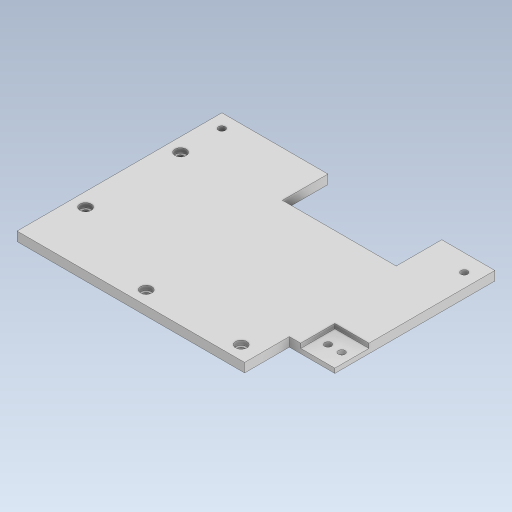
# Autodesk Inventor part: Casis Kanan Bawah
Saved by Autodesk Inventor 2023.5 (Build 275446000, 446)
## iProperties
Created: 2025-09-16
Part Number: Casis Kanan Bawah
Material: Generic
Document SubType Name: Modeling
Designer: Guntur
Density: 1 g/cm^3
Appearance: Default
Author: Guntur
Autodesk Inventor part; units mm, degrees
ref_plane "YZ Plane" through (0, 0, 0) normal (1, 0, 0) x (0, 1, 0)
ref_plane "XZ Plane" through (0, 0, 0) normal (0, 1, 0) x (-1, 0, 0)
ref_plane "XY Plane" through (0, 0, 0) normal (0, 0, 1) x (1, 0, 0)
sketch "Sketch1" plane through (0, 0, 0) normal (0, 1, 0) x (-1, 0, 0)
  circle A0 centre (-7.6905, 26.7159) radius 1.5
  circle A1 centre (-7.6905, 14.7159) radius 1.5
  line L0 (-0.1905, 5.7159) -> (-15.1905, 5.7159)
  line L1 (-15.1905, 35.7159) -> (-0.1905, 35.7159)
  line L2 (-15.1905, 5.7159) -> (-15.1905, 35.7159)
  circle A2 centre (5.6845, 41.7159) radius 1.5
  circle A3 centre (5.6845, 41.7159) radius 2.5
  line L3 (-2.528, 47.7159) -> (7.472, 47.7159)
  circle A4 centre (50.4345, -18.1591) radius 2.5
  circle A5 centre (50.4345, -36.2841) radius 1.5
  line L4 (9.8095, -42.2841) -> (9.8095, -22.2841)
  circle A6 centre (50.4345, -18.1591) radius 1.5
  line L5 (-0.1905, 35.7159) -> (-0.1905, 5.7159)
  line L6 (56.4345, 47.7159) -> (7.472, 47.7159)
  circle A7 centre (50.4345, 23.5909) radius 1.5
  line L7 (56.4345, -42.2841) -> (56.4345, 47.7159)
  line L8 (42.1595, 2.7159) -> (61.2095, 2.7159) construction
  circle A8 centre (50.4345, 23.5909) radius 2.5
  line L9 (-15.1905, 35.7159) -> (-30.1905, 35.7159)
  line L10 (-63.5655, 30.7159) -> (-63.5655, 47.7159)
  line L11 (-63.5655, 47.7159) -> (-48.5655, 47.7159)
  line L12 (-2.528, 47.7159) -> (-63.5655, 47.7159)
  circle A9 centre (-36.0655, 41.7159) radius 1.5
  circle A10 centre (-36.0655, 41.7159) radius 2.5
  circle A11 centre (-21.1905, -7.2841) radius 1.5
  line L13 (-27.6905, 2.7159) -> (-27.6905, -17.2841)
  circle A12 centre (-57.5655, -34.7841) radius 1.5
  line L14 (-2.6905, 2.7159) -> (-27.6905, 2.7159)
  circle A13 centre (-9.1905, -7.2841) radius 1.5
  line L15 (-2.6905, -17.2841) -> (-2.6905, 2.7159)
  line L16 (-27.6905, -17.2841) -> (-2.6905, -17.2841)
  line L17 (-63.5655, 47.7159) -> (-63.5655, -42.2841)
  line L18 (9.8095, -22.2841) -> (-40.1905, -22.2841)
  line L19 (-40.1905, -22.2841) -> (-40.1905, -42.2841)
  line L20 (-40.1905, -42.2841) -> (9.8095, -42.2841)
  line L21 (-63.5655, -42.2841) -> (56.4345, -42.2841)
  line L22 (-63.5655, 28.0659) -> (-48.5655, 28.0659)
  circle A14 centre (-22.6905, 26.7159) radius 1.5
  circle A15 centre (-53.0655, 20.5659) radius 1.5
  circle A16 centre (-59.0655, 20.5659) radius 1.5
  circle A17 centre (-53.0655, 20.5659) radius 2.5
  circle A18 centre (-22.6905, 14.7159) radius 1.5
  line L23 (-15.1905, 5.7159) -> (-15.1905, 35.7159)
  line L24 (-30.1905, 5.7159) -> (-15.1905, 5.7159)
  line L25 (-48.5655, 28.0659) -> (-48.5655, 13.0659)
  line L26 (-30.1905, 35.7159) -> (-30.1905, 5.7159)
  circle A19 centre (-59.0655, 20.5659) radius 2.5
  line L27 (-48.5655, 13.0659) -> (-63.5655, 13.0659)
  line L28 (-63.5655, 13.0659) -> (-63.5655, 28.0659)
  line L29 (-15.1905, 2.7159) -> (-15.1905, 34.925) construction
  line L30 (-48.5655, 28.0659) -> (-43.5655, 28.0659)
  line L31 (-43.5655, 28.0659) -> (-43.5655, 47.7159)
  point P0 (0, 0)
  point P1 (5.1035, 21.0043)
  point P2 (5.6845, 35.7159)
  point P3 (2.472, 2.7159)
  point P4 (-36.0655, 35.7159)
  point P5 (-2.6905, -7.2841)
  dimension "d4" = 12
  dimension "d5" = 7.5
  dimension "d6" = 12
  dimension "d7" = 9
  dimension "d8" = 0
  dimension "d10" = 0
  dimension "d11" = 5
  constraints: 64 end point, 20 centre point, 6 coincident, 2 point on line, 2 vertical, 1 horizontal, 1 midpoint, 1 perpendicular
  measures "d4" distance of A14.centre A18.centre
  measures "d5" distance from line of L26 A18.centre
  measures "d6" distance of A1.centre A0.centre
  measures "d7" distance from line of A0.centre L1
  measures "d8" distance between parallel lines of L29 L2
  measures "d10" distance between parallel lines of L29 L23
  measures "d11" distance of L22.end L30.end
extrude "Extrusion1" add sketch "Sketch1" along normal blind 4 contours A0 | A1 | L0 L2 L1 L5 | L24 L26 L9 L2 | L3 L6 L7 L21 L4 L18 L19 L17 L27 L25 L30 L31 L12 | A11 | L14 L15 L16 L13 | A13 | A14 | A18
extrude "Extrusion2" add sketch "Sketch1" along normal blind 2 contours L0 L2 L1 L5 | L24 L26 L9 L2 | A3 | L25 L27 L17 L22 | A4 | A8 | A10 | L14 L15 L16 L13 | A17 | A19
body "Solid1"
